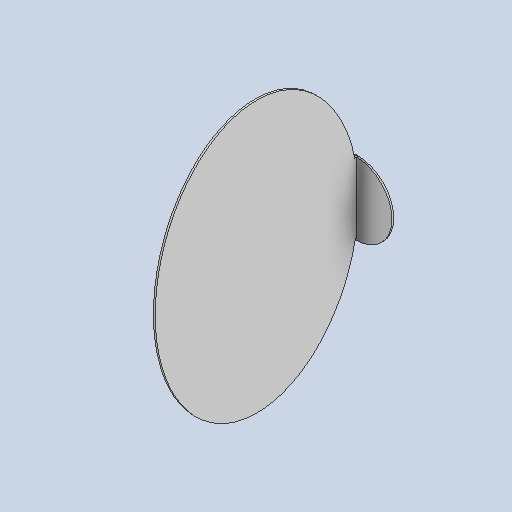
# Autodesk Inventor part: опорная окружность
Saved by Autodesk Inventor 2023.1 (Build 271208000, 208)
## iProperties
Created: 2024-11-21
Part Number: опорная окружность
Material: Типовые
Document SubType Name: Modeling
Designer: DELL
Density: 1 g/cm^3
Appearance: По умолчанию
Author: DELL
Autodesk Inventor part; units mm, degrees
ref_plane "YZ Plane" through (0, 0, 0) normal (1, 0, 0) x (0, 1, 0)
ref_plane "XZ Plane" through (0, 0, 0) normal (0, 1, 0) x (-1, 0, 0)
ref_plane "XY Plane" through (0, 0, 0) normal (0, 0, 1) x (1, 0, 0)
sketch "Эскиз1" plane through (0, 0, 0) normal (0, 0, 1) x (1, 0, 0)
  circle A0 centre (0, 0) radius 80 projected
  point P0 (0, 0)
extrude "Выдавливание1" add sketch "Эскиз1" along normal blind 4
sketch "Эскиз2" plane through (0, 0, 0) normal (1, 0, 0) x (0, 1, 0)
  line L0 (-300, 0) -> (300, 0) construction
  line L1 (300, 0) -> (300, 450) construction
  line L2 (300, 450) -> (-300, 450) construction
  line L3 (-300, 450) -> (-300, 0) construction
  line L4 (300, 450) -> (-300, 0) construction
  line L5 (0, 0) -> (0, 768.792) construction
  ellipse E0 centre (0, 225) end of major axis (-300, 225) minor radius 225 (80, 8.1475) -> (-75, 7.1447) ccw
  line L6 (80, 0) -> (-80, 0) projected
  line L7 (80, 0) -> (-75, 0)
  line L8 (-75, 0) -> (-75, 7.1447)
  line L9 (80, 8.1475) -> (80, 0)
  dimension "d2" = 450
  dimension "d3" = 600
  constraints: 18 end point, 3 parallel, 2 horizontal, 2 perpendicular, 1 coincident, 1 midpoint, 1 point on line, 1 vertical, 5 other
  measures "d2" distance of L2.end L0.start
  measures "d3" distance of L0.start L0.end
extrude "Выдавливание2" add sketch "Эскиз2" along normal mid plane 4
